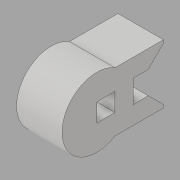
# Autodesk Inventor part: toggleLatch
Saved by Autodesk Inventor 2017 (Build 210142000, 142)
## iProperties
Created: 2019-05-14
Part Number: toggleLatch
Material: Generic
Document SubType Name: Modeling
Designer: Joe Sedutto
Density: 1 g/cm^3
Appearance: Default
Author: Joe Sedutto
Autodesk Inventor part; units mm, degrees
ref_plane "YZ Plane" through (0, 0, 0) normal (1, 0, 0) x (0, 1, 0)
ref_plane "XZ Plane" through (0, 0, 0) normal (0, 1, 0) x (-1, 0, 0)
ref_plane "XY Plane" through (0, 0, 0) normal (0, 0, 1) x (1, 0, 0)
sketch "Sketch1" plane through (0, 0, 0) normal (1, 0, 0) x (0, 1, 0)
  line L0 (0, 0) -> (3.048, 0)
  line L1 (3.048, 0) -> (3.048, 5.08)
  line L2 (3.048, 5.08) -> (0, 5.08)
  line L3 (0, 5.08) -> (0, 0)
  line L4 (0, 5.08) -> (9.906, 5.08)
  line L5 (9.906, 5.08) -> (9.906, 8.128)
  line L6 (9.906, 8.128) -> (0, 8.128)
  line L7 (0, 8.128) -> (0, 5.08)
  line L8 (9.906, 5.08) -> (6.858, 5.08)
  line L9 (6.858, 5.08) -> (6.858, 0)
  line L10 (6.858, 0) -> (9.906, 0)
  line L11 (9.906, 0) -> (9.906, 5.08)
  dimension "d0" = 3.048
  dimension "d1" = 5.08
  dimension "d3" = 3.048
  dimension "d4" = 3.81
  constraints: 24 end point, 6 parallel, 3 horizontal, 3 perpendicular, 2 equal length
  measures "d0" distance of L2.end L1.end
  measures "d1" distance of L1.end L0.end
  measures "d3" distance of L5.end L4.end
  measures "d4" distance between parallel lines of L1 L9
extrude "Extrusion1" add sketch "Sketch1" along normal blind 7.62
sketch "Sketch2" plane through (7.62, 0, 0) normal (1, 0, 0) x (0, 0, -1)
  line L0 (-11.176, 6.477) -> (-8.128, 6.477)
  line L1 (-8.128, 6.477) -> (-8.128, 3.429)
  line L2 (-8.128, 3.429) -> (-11.176, 3.429)
  line L3 (-11.176, 3.429) -> (-11.176, 6.477)
  line L4 (-8.128, 9.906) -> (-8.128, 0) projected
  circle A0 centre (-11.176, 4.953) radius 5.8157
  point P0 (0, 0)
  point P1 (-8.128, 4.953)
  point P2 (-11.176, 4.953)
  dimension "d7" = 3.048
  constraints: 8 end point, 3 midpoint, 2 parallel, 2 perpendicular, 2 point on circle, 1 centre point, 1 coincident, 1 horizontal
  measures "d7" distance of L0.start L0.end
extrude "Extrusion2" add sketch "Sketch2" against normal blind 7.62 contours L3 L2 L4 A0 L0
chamfer "Chamfer1" distance 2.54 angle 45 2 edges at (3.81, 3.048, 0) (3.81, 6.858, 0)
body "Solid1"
